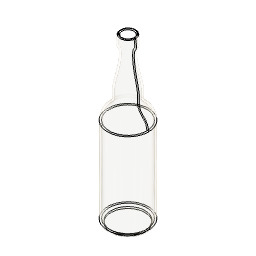
Tutorial 2 Soda Bottle v5 (Autodesk Fusion 360 design; units mm, degrees)
Autodesk Fusion 360 part; units mm, degrees
sketch "Sketch1" plane through (0, 0, 0) normal (0, 1, 0) x (1, 0, 0) in component "Bottle"
  line L0 (0, 0) -> (0, -239.9714)
  line L1 (0, 0) -> (30, 0)
  line L2 (30, 0) -> (30, -130)
  spline S0 degree 5 poles (30, -130) (30, -130.6436) (29.9681, -131.9089) (29.8248, -133.7408) (29.4321, -136.0503) (28.5606, -138.713) (27.2789, -141.1591) (25.6037, -143.413) (23.6384, -145.5265) (21.5839, -147.5806) (19.6753, -149.6669) (18.1284, -151.8721) (17.0893, -154.2627) (16.5664, -156.8654) (16.4441, -159.6723) (16.5407, -162.6621) (16.6531, -165.816) (16.6057, -169.1351) (16.3012, -172.6597) (15.7117, -176.4525) (14.8637, -180.5776) (13.8246, -185.0812) (12.6896, -189.9721) (11.5681, -195.2002) (10.5721, -200.6388) (9.7979, -206.0573) (9.3082, -211.1643) (9.1359, -215.6662) (9.2805, -219.3199) (9.7073, -221.9901) (10.3458, -223.7001) (11.0863, -224.6985) (11.7825, -225.4865) (12.2925, -226.605) (12.5204, -228.4239) (12.4111, -231.1565) (12.0325, -234.1575) (11.5812, -236.8809) (11.2061, -238.9063) (11, -239.9714) knots 0 0 0 0 0 0 0.028571 0.057143 0.085714 0.114286 0.142857 0.171429 0.2 0.228571 0.257143 0.285714 0.314286 0.342857 0.371429 0.4 0.428571 0.457143 0.485714 0.514286 0.542857 0.571429 0.6 0.628571 0.657143 0.685714 0.714286 0.742857 0.771429 0.8 0.828571 0.857143 0.885714 0.914286 0.942857 0.971429 1 1 1 1 1 1
  line L3 (14.2878, -181.2079) -> (8.5255, -211.2771)
  line L4 (30, -116.8953) -> (30, -143.1047)
  line L5 (0, -239.9714) -> (11, -239.9714)
  point P0 (26.0306, -142.7547)
  point P1 (17.8171, -152.7711)
  point P2 (16.6152, -166.1932)
  point P3 (11.4066, -196.2425)
  point P4 (10.2824, -223.3357)
  point P5 (11.8073, -225.6908)
  dimension "d1" = 130
  dimension "d5" = 11
  constraint coincident L0.start L1.start
  constraint vertical L0
  constraint perpendicular L0 L1
  constraint perpendicular L1 L2
  constraint midpoint P3 L3
  constraint midpoint L2.end L4
  constraint vertical L4
  constraint horizontal L5
  measures "d1" distance of L1.end L2.end
  measures "d5" distance of L0.end S0.end
revolve "Revolve1" add sketch "Sketch1" angle 360 about axis through (0, 0, 0) along (0, 0, 1)
fillet "Fillet1" radius 5 1 edges at (-27.9698, -10.8485, 0)
shell "Shell1" thickness 2.5 removed faces 1 at (-3.2467, -0.051, 239.9714)
fillet "Fillet2" radius 1 1 edges at (-8.4536, 0.0033, 239.9714)
fillet "Fillet3" radius 1 1 edges at (-10.2556, -3.9778, 239.9714)
component "Bottle" placed x (1, 0, 0) y (0, 1, 0) z (0, 0, 1) at (0, 0, 0)
